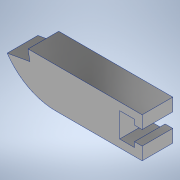
# Autodesk Inventor part: Finray_test_8_Kerbe_10deg
Saved by Autodesk Inventor 2022 (Build 260153000, 153)
## iProperties
Created: 2022-02-28
Part Number: Finray_test_8_Kerbe_10deg
Material: Generic
Document SubType Name: Modeling
Designer: richa
Density: 1 g/cm^3
Appearance: Aluminum - Flat
Author: richa
Autodesk Inventor part; units mm, degrees
ref_plane "YZ Plane" through (0, 0, 0) normal (1, 0, 0) x (0, 1, 0)
ref_plane "XZ Plane" through (0, 0, 0) normal (0, 1, 0) x (-1, 0, 0)
ref_plane "XY Plane" through (0, 0, 0) normal (0, 0, 1) x (1, 0, 0)
sketch "Sketch5" plane through (0, 0, 0) normal (0, 0, 1) x (1, 0, 0)
  line L0 (52.8, -15.6) -> (52.8, -10.6)
  line L1 (52.8, -10.6) -> (49.8, -10.6)
  line L2 (49.8, -10.6) -> (49.8, -12.6)
  line L3 (44, -12.6) -> (44, -3)
  line L4 (49.8, -3) -> (49.8, -5)
  line L5 (49.8, -5) -> (52.8, -5)
  line L6 (52.8, -5) -> (52.8, 0)
  line L7 (52.8, 0) -> (7.8, 0)
  line L8 (44, -3) -> (49.8, -3)
  line L9 (44, -12.6) -> (49.8, -12.6)
  line L10 (52.8, -15.6) -> (7.8, -15.6)
  line L11 (7.8, -15.6) -> (0, -15.6)
  line L12 (0, -15.6) -> (0, 0)
  line L13 (0, 0) -> (7.8, 0)
  point P0 (7.8, 0)
  dimension "d41" = 5.8
  dimension "d48" = 44
  dimension "d50" = 3
  dimension "d63" = 45
  dimension "d71" = 0
  dimension "d87" = 5.6
  dimension "d88" = 9.6
  dimension "d97" = 15.6
  constraints: 28 end point, 8 perpendicular, 4 collinear, 3 parallel, 2 horizontal, 1 vertical
  measures "d41" distance between parallel lines of L2 L3
  measures "d48" distance from line of L3 L12.end
  measures "d50" distance of L4.end L5.end
  measures "d63" distance of L0.start L10.end
  measures "d71" distance from line of L12.end L7
  measures "d87" distance from line of L0.end L5
  measures "d88" distance of L3.start L3.end
  measures "d97" distance of L11.end L12.end
extrude "Extrusion2" add sketch "Sketch5" along normal blind 12
sketch "Sketch8" plane through (0, 0, 0) normal (0, 0, -1) x (-1, 0, 0)
  line L0 (-8.1687, 0) -> (-8.8633, -3.9392)
  line L1 (-7.8, 0) -> (-1.143, 0) construction
  line L2 (0, -5.5021) -> (-8.8633, -3.9392)
  line L3 (-7.8, 0) -> (-8.1687, 0)
  line L4 (0, 0) -> (0, -15.6) projected
  line L5 (-52.8, 0) -> (0, 0) projected
  line L6 (-7.8, 0) -> (0, 0)
  line L7 (0, 0) -> (0, -5.5021)
  dimension "d80" = 100
  dimension "d95" = 4
  dimension "d96" = 9
  constraints: 12 end point, 2 collinear, 2 perpendicular, 1 horizontal, 1 point on line
  measures "d80" angle of L0 L1
  measures "d95" distance of L0.start L0.end
  measures "d96" distance of L2.start L0.end
extrude "Extrusion5" cut sketch "Sketch8" against normal through all
fillet "Fillet2" radius 23 1 edges at (0, -15.6, 6)
equation "\"l1\" = 8"
body "Solid2"
